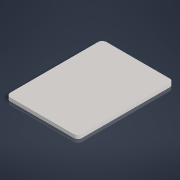
# Autodesk Inventor part: Stand_plate
Saved by Autodesk Inventor 2022 (Build 260153070, 153G)
## iProperties
Created: 2021-12-15
Part Number: Stand_plate
Material: Типовые
Document SubType Name: Modeling
Designer: kalugin_a
Density: 1 g/cm^3
Appearance: По умолчанию
Author: kalugin_a
Autodesk Inventor part; units mm, degrees
ref_plane "YZ Plane" through (0, 0, 0) normal (1, 0, 0) x (0, 1, 0)
ref_plane "XZ Plane" through (0, 0, 0) normal (0, 1, 0) x (-1, 0, 0)
ref_plane "XY Plane" through (0, 0, 0) normal (0, 0, 1) x (1, 0, 0)
sketch "Эскиз1" plane through (0, 0, 0) normal (0, 1, 0) x (-1, 0, 0)
  line L0 (-128.6249, -74.7454) -> (162.1285, -74.7454)
  line L1 (182.1285, -94.7454) -> (182.1285, -498.4111)
  line L2 (162.1285, -518.4111) -> (-128.6249, -518.4111)
  line L3 (-148.6249, -498.4111) -> (-148.6249, -94.7454)
  arc A0 (182.1285, -76.7454) -> (180.1285, -74.7454) centre (180.1285, -76.7454) ccw
  arc A1 (182.1285, -94.7454) -> (162.1285, -74.7454) centre (162.1285, -94.7454) ccw
  arc A2 (-128.6249, -74.7454) -> (-148.6249, -94.7454) centre (-128.6249, -94.7454) ccw
  arc A3 (-148.6249, -498.4111) -> (-128.6249, -518.4111) centre (-128.6249, -498.4111) ccw
  arc A4 (162.1285, -518.4111) -> (182.1285, -498.4111) centre (162.1285, -498.4111) ccw
  dimension "d0" = 2
  dimension "d1" = 20
  constraints: 10 point on circle, 10 tangent, 8 end point, 5 centre point, 3 equal radius, 2 parallel, 2 point on line, 1 horizontal, 1 perpendicular
  measures "d0" radius of A0
  measures "d1" radius of A1
extrude "Выдавливание1" add sketch "Эскиз1" along normal blind 16
